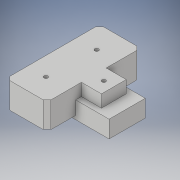
# Autodesk Inventor part: Connect_Male_Beauty
Saved by Autodesk Inventor 2019 (Build 230136000, 136)
## iProperties
Created: 2020-03-28
Part Number: Connect_Male_Beauty
Material: Generico
Document SubType Name: Modeling
Designer: Administrator
Density: 1 g/cm^3
Appearance: Default
Author: Administrator
Autodesk Inventor part; units mm, degrees
ref_plane "YZ Plane" through (0, 0, 0) normal (1, 0, 0) x (0, 1, 0)
ref_plane "XZ Plane" through (0, 0, 0) normal (0, 1, 0) x (-1, 0, 0)
ref_plane "XY Plane" through (0, 0, 0) normal (0, 0, 1) x (1, 0, 0)
sketch "Sketch1" plane through (0, 0, 0) normal (0, 1, 0) x (-1, 0, 0)
  line L0 (0, 0) -> (-17.5, 0)
  line L1 (-17.5, 0) -> (-17.5, -19)
  line L2 (-17.5, -19) -> (0, -19)
  line L3 (0, -19) -> (0, 0)
  dimension "d0" = 17.5
  dimension "d1" = 19
  constraints: 8 end point, 2 parallel, 1 horizontal, 1 perpendicular
  measures "d0" distance of L2.end L1.end
  measures "d1" distance of L1.end L0.end
extrude "Extrusion1" add sketch "Sketch1" along normal blind 9
sketch "Sketch2" plane through (0, 9, 0) normal (0, 1, 0) x (1, 0, 0)
  line L0 (0, 3) -> (10.5, 3)
  line L1 (10.5, 3) -> (10.5, 16)
  line L2 (10.5, 16) -> (0, 16)
  line L3 (0, 16) -> (0, 3)
  point P0 (0, 0)
  dimension "d4" = 10.5
  dimension "d5" = 13
  constraints: 8 end point, 2 parallel, 1 horizontal, 1 perpendicular
  measures "d4" distance of L2.end L1.end
  measures "d5" distance of L1.end L0.end
extrude "Extrusion2" add sketch "Sketch2" along normal blind 3
sketch "Sketch3" plane through (0, 0, -19) normal (-1, 0, 0) x (0, 0, 1)
  line L0 (18.2159, 3.93) -> (-8.9493, 3.93) construction
  line L1 (-8.9493, 3.93) -> (-8.9493, 7.5955) construction
  line L2 (-8.9493, 7.5955) -> (18.2159, 7.5955) construction
  line L3 (18.2159, 7.5955) -> (18.2159, 3.93) construction
  spline S0 degree 2 poles (15.88, 5.4433) (15.88, 5.6763) (15.9813, 6.1119) (16.0766, 6.2922) knots 0 0 0 1 2 2 2
  line L4 (16.0766, 6.2922) -> (16.6418, 6.2922)
  line L5 (16.6418, 6.2922) -> (16.6762, 6.0977)
  spline S1 degree 2 poles (16.6762, 6.0977) (16.7654, 6.1929) (16.9173, 6.3064) (17.049, 6.3064) knots 0 0 0 1 2 2 2
  spline S2 degree 2 poles (17.049, 6.3064) (17.2556, 6.3064) (17.519, 5.8911) (17.519, 5.498) knots 0 0 0 1 2 2 2
  spline S3 degree 2 poles (17.519, 5.498) (17.519, 5.103) (17.1949, 4.6634) (16.9882, 4.6634) knots 0 0 0 1 2 2 2
  spline S4 degree 2 poles (16.9882, 4.6634) (16.891, 4.6634) (16.7512, 4.7241) (16.6803, 4.7748) knots 0 0 0 1 2 2 2
  line L6 (16.6803, 4.7748) -> (16.6803, 4.6937)
  line L7 (16.6803, 4.6937) -> (16.4655, 4.6937)
  line L8 (16.4655, 4.6937) -> (16.4655, 6.1058)
  line L9 (16.4655, 6.1058) -> (16.1596, 6.1058)
  spline S5 degree 2 poles (16.1596, 6.1058) (16.109, 5.9863) (16.0644, 5.6074) (16.0644, 5.4535) knots 0 0 0 1 2 2 2
  spline S6 degree 2 poles (16.0644, 5.4535) (16.0644, 4.9044) (16.5121, 4.2359) (16.9315, 4.2359) knots 0 0 0 1 2 2 2
  spline S7 degree 2 poles (16.9315, 4.2359) (17.3286, 4.2359) (17.8472, 4.9591) (17.8472, 5.4758) knots 0 0 0 1 2 2 2
  spline S8 degree 2 poles (17.8472, 5.4758) (17.8472, 6.0288) (17.3448, 6.7156) (16.9396, 6.7156) knots 0 0 0 1 2 2 2
  spline S9 degree 2 poles (16.9396, 6.7156) (16.8302, 6.7156) (16.5891, 6.6792) (16.4817, 6.6386) knots 0 0 0 1 2 2 2
  line L10 (16.4817, 6.6386) -> (16.4817, 6.8757)
  spline S10 degree 2 poles (16.4817, 6.8757) (16.5952, 6.9101) (16.8282, 6.9364) (16.9396, 6.9364) knots 0 0 0 1 2 2 2
  spline S11 degree 2 poles (16.9396, 6.9364) (17.4157, 6.9364) (18.0397, 6.12) (18.0397, 5.4717) knots 0 0 0 1 2 2 2
  spline S12 degree 2 poles (18.0397, 5.4717) (18.0397, 4.8558) (17.3954, 4.009) (16.9335, 4.009) knots 0 0 0 1 2 2 2
  spline S13 degree 2 poles (16.9335, 4.009) (16.4392, 4.009) (15.88, 4.8052) (15.88, 5.4433) knots 0 0 0 1 2 2 2
  line L11 (16.6823, 5.8728) -> (16.6823, 5.0037)
  spline S14 degree 2 poles (16.6823, 5.0037) (16.7573, 4.9551) (16.8849, 4.9125) (16.9518, 4.9125) knots 0 0 0 1 2 2 2
  spline S15 degree 2 poles (16.9518, 4.9125) (17.1037, 4.9125) (17.2901, 5.1962) (17.2901, 5.494) knots 0 0 0 1 2 2 2
  spline S16 degree 2 poles (17.2901, 5.494) (17.2901, 5.7614) (17.1503, 6.0471) (16.9963, 6.0471) knots 0 0 0 1 2 2 2
  spline S17 degree 2 poles (16.9963, 6.0471) (16.9153, 6.0471) (16.7552, 5.9498) (16.6823, 5.8728) knots 0 0 0 1 2 2 2
  line L12 (15.7301, 6.5576) -> (15.0555, 4.0576)
  line L13 (15.0555, 4.0576) -> (14.7273, 4.0576)
  line L14 (14.7273, 4.0576) -> (14.0527, 6.5576)
  line L15 (14.0527, 6.5576) -> (14.3322, 6.5576)
  line L16 (14.3322, 6.5576) -> (14.5125, 5.8587)
  line L17 (14.5125, 5.8587) -> (15.2804, 5.8587)
  line L18 (15.2804, 5.8587) -> (15.4607, 6.5576)
  line L19 (15.4607, 6.5576) -> (15.7301, 6.5576)
  line L20 (14.5875, 5.575) -> (14.8975, 4.3919)
  line L21 (14.8975, 4.3919) -> (15.2054, 5.575)
  line L22 (15.2054, 5.575) -> (14.5875, 5.575)
  spline S18 degree 2 poles (13.1106, 5.9073) (13.1106, 6.2355) (13.4307, 6.592) (13.7022, 6.592) knots 0 0 0 1 2 2 2
  spline S19 degree 2 poles (13.7022, 6.592) (13.765, 6.592) (13.9817, 6.5637) (14.0547, 6.5434) knots 0 0 0 1 2 2 2
  line L23 (14.0547, 6.5434) -> (14.0547, 6.2233)
  line L24 (14.0547, 6.2233) -> (14.0405, 6.2233)
  spline S20 degree 2 poles (14.0405, 6.2233) (13.9838, 6.2476) (13.8217, 6.3044) (13.7366, 6.3044) knots 0 0 0 1 2 2 2
  spline S21 degree 2 poles (13.7366, 6.3044) (13.613, 6.3044) (13.4672, 6.2334) (13.4327, 6.1686) knots 0 0 0 1 2 2 2
  spline S22 degree 2 poles (13.4327, 6.1686) (13.3962, 6.1018) (13.376, 5.9073) (13.376, 5.7796) knots 0 0 0 1 2 2 2
  line L25 (13.376, 5.7796) -> (13.376, 4.323)
  line L26 (13.376, 4.323) -> (13.7994, 4.323)
  line L27 (13.7994, 4.323) -> (13.7994, 4.0576)
  line L28 (13.7994, 4.0576) -> (13.1106, 4.0576)
  line L29 (13.1106, 4.0576) -> (13.1106, 5.9073)
  spline S23 degree 2 poles (12.0206, 6.6103) (12.1969, 6.6103) (12.4603, 6.4948) (12.5535, 6.3793) knots 0 0 0 1 2 2 2
  spline S24 degree 2 poles (12.5535, 6.3793) (12.6588, 6.2497) (12.7439, 5.885) (12.7439, 5.6176) knots 0 0 0 1 2 2 2
  line L30 (12.7439, 5.6176) -> (12.7439, 4.0576)
  line L31 (12.7439, 4.0576) -> (12.4785, 4.0576)
  line L32 (12.4785, 4.0576) -> (12.4785, 5.6176)
  spline S25 degree 2 poles (12.4785, 5.6176) (12.4785, 5.7918) (12.4441, 6.0268) (12.3934, 6.122) knots 0 0 0 1 2 2 2
  spline S26 degree 2 poles (12.3934, 6.122) (12.3387, 6.2233) (12.1544, 6.3266) (12.0206, 6.3266) knots 0 0 0 1 2 2 2
  spline S27 degree 2 poles (12.0206, 6.3266) (11.8971, 6.3266) (11.7026, 6.2233) (11.6479, 6.122) knots 0 0 0 1 2 2 2
  spline S28 degree 2 poles (11.6479, 6.122) (11.5992, 6.0268) (11.5628, 5.7938) (11.5628, 5.6257) knots 0 0 0 1 2 2 2
  line L33 (11.5628, 5.6257) -> (11.5628, 4.0576)
  line L34 (11.5628, 4.0576) -> (11.2974, 4.0576)
  line L35 (11.2974, 4.0576) -> (11.2974, 5.6176)
  spline S29 degree 2 poles (11.2974, 5.6176) (11.2974, 5.8789) (11.3825, 6.2517) (11.4878, 6.3793) knots 0 0 0 1 2 2 2
  spline S30 degree 2 poles (11.4878, 6.3793) (11.583, 6.4968) (11.8363, 6.6103) (12.0206, 6.6103) knots 0 0 0 1 2 2 2
  spline S31 degree 2 poles (10.3594, 6.6022) (10.5762, 6.6022) (10.8821, 6.4887) (11.0158, 6.4077) knots 0 0 0 1 2 2 2
  line L36 (11.0158, 6.4077) -> (11.0158, 5.9903)
  line L37 (11.0158, 5.9903) -> (10.9975, 5.9903)
  spline S32 degree 2 poles (10.9975, 5.9903) (10.8659, 6.1443) (10.5316, 6.3145) (10.3776, 6.3145) knots 0 0 0 1 2 2 2
  spline S33 degree 2 poles (10.3776, 6.3145) (10.1568, 6.3145) (9.9319, 6.0856) (9.9319, 5.8971) knots 0 0 0 1 2 2 2
  spline S34 degree 2 poles (9.9319, 5.8971) (9.9319, 5.7472) (10.0514, 5.5608) (10.1791, 5.5142) knots 0 0 0 1 2 2 2
  spline S35 degree 2 poles (10.1791, 5.5142) (10.2723, 5.4818) (10.4262, 5.4373) (10.5417, 5.4008) knots 0 0 0 1 2 2 2
  spline S36 degree 2 poles (10.5417, 5.4008) (10.645, 5.3664) (10.8091, 5.263) (10.8719, 5.18) knots 0 0 0 1 2 2 2
  spline S37 degree 2 poles (10.8719, 5.18) (10.9327, 5.0969) (11.0016, 4.874) (11.0016, 4.7282) knots 0 0 0 1 2 2 2
  spline S38 degree 2 poles (11.0016, 4.7282) (11.0016, 4.4243) (10.6227, 4.013) (10.329, 4.013) knots 0 0 0 1 2 2 2
  spline S39 degree 2 poles (10.329, 4.013) (10.1608, 4.013) (9.861, 4.0961) (9.7334, 4.1751) knots 0 0 0 1 2 2 2
  line L38 (9.7334, 4.1751) -> (9.7334, 4.5722)
  line L39 (9.7334, 4.5722) -> (9.7536, 4.5722)
  spline S40 degree 2 poles (9.7536, 4.5722) (9.8488, 4.4628) (10.1467, 4.3007) (10.3108, 4.3007) knots 0 0 0 1 2 2 2
  spline S41 degree 2 poles (10.3108, 4.3007) (10.4971, 4.3007) (10.7261, 4.5175) (10.7261, 4.6937) knots 0 0 0 1 2 2 2
  spline S42 degree 2 poles (10.7261, 4.6937) (10.7261, 4.8518) (10.5903, 5.0402) (10.4627, 5.0827) knots 0 0 0 1 2 2 2
  spline S43 degree 2 poles (10.4627, 5.0827) (10.3796, 5.1111) (10.1345, 5.184) (10.0535, 5.2144) knots 0 0 0 1 2 2 2
  spline S44 degree 2 poles (10.0535, 5.2144) (9.8468, 5.2934) (9.6564, 5.6115) (9.6564, 5.8445) knots 0 0 0 1 2 2 2
  spline S45 degree 2 poles (9.6564, 5.8445) (9.6564, 5.9924) (9.7516, 6.276) (9.8367, 6.3753) knots 0 0 0 1 2 2 2
  spline S46 degree 2 poles (9.8367, 6.3753) (9.9339, 6.4847) (10.177, 6.6022) (10.3594, 6.6022) knots 0 0 0 1 2 2 2
  spline S47 degree 2 poles (8.1714, 5.6196) (8.1714, 6.0937) (8.536, 6.6103) (8.8399, 6.6103) knots 0 0 0 1 2 2 2
  spline S48 degree 2 poles (8.8399, 6.6103) (9.1519, 6.6103) (9.5105, 6.0775) (9.5105, 5.6196) knots 0 0 0 1 2 2 2
  spline S49 degree 2 poles (9.5105, 5.6196) (9.5105, 5.1496) (9.1418, 4.6289) (8.8399, 4.6289) knots 0 0 0 1 2 2 2
  spline S50 degree 2 poles (8.8399, 4.6289) (8.536, 4.6289) (8.1714, 5.1475) (8.1714, 5.6196) knots 0 0 0 1 2 2 2
  spline S51 degree 2 poles (8.4327, 5.6196) (8.4327, 5.2549) (8.6434, 4.9004) (8.8399, 4.9004) knots 0 0 0 1 2 2 2
  spline S52 degree 2 poles (8.8399, 4.9004) (9.0364, 4.9004) (9.2492, 5.2549) (9.2492, 5.6196) knots 0 0 0 1 2 2 2
  spline S53 degree 2 poles (9.2492, 5.6196) (9.2492, 5.9741) (9.0364, 6.3388) (8.8399, 6.3388) knots 0 0 0 1 2 2 2
  spline S54 degree 2 poles (8.8399, 6.3388) (8.6454, 6.3388) (8.4327, 5.9802) (8.4327, 5.6196) knots 0 0 0 1 2 2 2
  line L40 (7.124, 4.2501) -> (7.1381, 4.2501)
  spline S55 degree 2 poles (7.1381, 4.2501) (7.1706, 4.2339) (7.2962, 4.2055) (7.3468, 4.2055) knots 0 0 0 1 2 2 2
  spline S56 degree 2 poles (7.3468, 4.2055) (7.5048, 4.2055) (7.6406, 4.3838) (7.6406, 4.6188) knots 0 0 0 1 2 2 2
  line L41 (7.6406, 4.6188) -> (7.6406, 4.6816)
  line L42 (7.6406, 4.6816) -> (7.2253, 4.6816)
  line L43 (7.2253, 4.6816) -> (7.2253, 4.9429)
  line L44 (7.2253, 4.9429) -> (7.6325, 4.9429)
  line L45 (7.6325, 4.9429) -> (7.6325, 6.5576)
  line L46 (7.6325, 6.5576) -> (7.8857, 6.5576)
  line L47 (7.8857, 6.5576) -> (7.8857, 4.9429)
  line L48 (7.8857, 4.9429) -> (8.0559, 4.9429)
  line L49 (8.0559, 4.9429) -> (8.0559, 4.6816)
  line L50 (8.0559, 4.6816) -> (7.8857, 4.6816)
  line L51 (7.8857, 4.6816) -> (7.8857, 4.6188)
  spline S57 degree 2 poles (7.8857, 4.6188) (7.8857, 4.2825) (7.6264, 3.93) (7.3833, 3.93) knots 0 0 0 1 2 2 2
  spline S58 degree 2 poles (7.3833, 3.93) (7.3124, 3.93) (7.1787, 3.9482) (7.124, 3.9604) knots 0 0 0 1 2 2 2
  line L52 (7.124, 3.9604) -> (7.124, 4.2501)
  spline S59 degree 2 poles (6.583, 6.5941) (6.7897, 6.5941) (7.0206, 6.3003) (7.0206, 5.9822) knots 0 0 0 1 2 2 2
  line L53 (7.0206, 5.9822) -> (7.0206, 4.9429)
  line L54 (7.0206, 4.9429) -> (7.1908, 4.9429)
  line L55 (7.1908, 4.9429) -> (7.1908, 4.6816)
  line L56 (7.1908, 4.6816) -> (7.0206, 4.6816)
  line L57 (7.0206, 4.6816) -> (7.0206, 4.1427)
  line L58 (7.0206, 4.1427) -> (6.7674, 4.1427)
  line L59 (6.7674, 4.1427) -> (6.7674, 4.6816)
  line L60 (6.7674, 4.6816) -> (6.3035, 4.6816)
  line L61 (6.3035, 4.6816) -> (6.3035, 4.9429)
  line L62 (6.3035, 4.9429) -> (6.7674, 4.9429)
  line L63 (6.7674, 4.9429) -> (6.7674, 5.8364)
  spline S60 degree 2 poles (6.7674, 5.8364) (6.7674, 5.9782) (6.7593, 6.1342) (6.733, 6.201) knots 0 0 0 1 2 2 2
  spline S61 degree 2 poles (6.733, 6.201) (6.7107, 6.2598) (6.6074, 6.3185) (6.5202, 6.3185) knots 0 0 0 1 2 2 2
  spline S62 degree 2 poles (6.5202, 6.3185) (6.4595, 6.3185) (6.344, 6.2719) (6.3176, 6.2578) knots 0 0 0 1 2 2 2
  line L64 (6.3176, 6.2578) -> (6.3035, 6.2578)
  line L65 (6.3035, 6.2578) -> (6.3035, 6.5414)
  spline S63 degree 2 poles (6.3035, 6.5414) (6.3744, 6.5657) (6.5202, 6.5941) (6.583, 6.5941) knots 0 0 0 1 2 2 2
  line L66 (5.724, 6.5576) -> (6.0441, 6.5576)
  line L67 (6.0441, 6.5576) -> (6.0441, 6.0795)
  line L68 (6.0441, 6.0795) -> (5.724, 6.0795)
  line L69 (5.724, 6.0795) -> (5.724, 6.5576)
  spline S64 degree 2 poles (4.6888, 6.6001) (4.8428, 6.6001) (5.1001, 6.4806) (5.1933, 6.3591) knots 0 0 0 1 2 2 2
  spline S65 degree 2 poles (5.1933, 6.3591) (5.2864, 6.2395) (5.3877, 5.8708) (5.3877, 5.6236) knots 0 0 0 1 2 2 2
  spline S66 degree 2 poles (5.3877, 5.6236) (5.3877, 5.3765) (5.2824, 5.0159) (5.1933, 4.8943) knots 0 0 0 1 2 2 2
  spline S67 degree 2 poles (5.1933, 4.8943) (5.1041, 4.7707) (4.8407, 4.639) (4.6888, 4.639) knots 0 0 0 1 2 2 2
  spline S68 degree 2 poles (4.6888, 4.639) (4.5652, 4.639) (4.3343, 4.7262) (4.2451, 4.7829) knots 0 0 0 1 2 2 2
  line L70 (4.2451, 4.7829) -> (4.2451, 5.1374)
  line L71 (4.2451, 5.1374) -> (4.2593, 5.1374)
  spline S69 degree 2 poles (4.2593, 5.1374) (4.2877, 5.1091) (4.3707, 5.0361) (4.4315, 4.9976) knots 0 0 0 1 2 2 2
  spline S70 degree 2 poles (4.4315, 4.9976) (4.4842, 4.9652) (4.626, 4.9146) (4.6928, 4.9146) knots 0 0 0 1 2 2 2
  spline S71 degree 2 poles (4.6928, 4.9146) (4.8894, 4.9146) (5.1264, 5.2853) (5.1264, 5.6236) knots 0 0 0 1 2 2 2
  spline S72 degree 2 poles (5.1264, 5.6236) (5.1264, 5.9539) (4.8975, 6.3246) (4.6928, 6.3246) knots 0 0 0 1 2 2 2
  spline S73 degree 2 poles (4.6928, 6.3246) (4.5693, 6.3246) (4.3464, 6.197) (4.2593, 6.0977) knots 0 0 0 1 2 2 2
  line L72 (4.2593, 6.0977) -> (4.2451, 6.0977)
  line L73 (4.2451, 6.0977) -> (4.2451, 6.4522)
  spline S74 degree 2 poles (4.2451, 6.4522) (4.2836, 6.4745) (4.395, 6.5373) (4.4416, 6.5515) knots 0 0 0 1 2 2 2
  spline S75 degree 2 poles (4.4416, 6.5515) (4.5065, 6.5758) (4.6078, 6.6001) (4.6888, 6.6001) knots 0 0 0 1 2 2 2
  spline S76 degree 2 poles (2.7824, 5.6196) (2.7824, 6.0937) (3.1471, 6.6103) (3.4509, 6.6103) knots 0 0 0 1 2 2 2
  spline S77 degree 2 poles (3.4509, 6.6103) (3.7629, 6.6103) (4.1215, 6.0775) (4.1215, 5.6196) knots 0 0 0 1 2 2 2
  spline S78 degree 2 poles (4.1215, 5.6196) (4.1215, 5.1496) (3.7528, 4.6289) (3.4509, 4.6289) knots 0 0 0 1 2 2 2
  spline S79 degree 2 poles (3.4509, 4.6289) (3.1471, 4.6289) (2.7824, 5.1475) (2.7824, 5.6196) knots 0 0 0 1 2 2 2
  spline S80 degree 2 poles (3.0437, 5.6196) (3.0437, 5.2549) (3.2544, 4.9004) (3.4509, 4.9004) knots 0 0 0 1 2 2 2
  spline S81 degree 2 poles (3.4509, 4.9004) (3.6475, 4.9004) (3.8602, 5.2549) (3.8602, 5.6196) knots 0 0 0 1 2 2 2
  spline S82 degree 2 poles (3.8602, 5.6196) (3.8602, 5.9741) (3.6475, 6.3388) (3.4509, 6.3388) knots 0 0 0 1 2 2 2
  spline S83 degree 2 poles (3.4509, 6.3388) (3.2565, 6.3388) (3.0437, 5.9802) (3.0437, 5.6196) knots 0 0 0 1 2 2 2
  line L74 (0.8213, 6.5576) -> (0.8213, 5.4717)
  spline S84 degree 2 poles (0.8213, 5.4717) (0.8213, 5.342) (0.8375, 5.1212) (0.8618, 5.0604) knots 0 0 0 1 2 2 2
  spline S85 degree 2 poles (0.8618, 5.0604) (0.8902, 4.9936) (0.9894, 4.9287) (1.0725, 4.9287) knots 0 0 0 1 2 2 2
  spline S86 degree 2 poles (1.0725, 4.9287) (1.1515, 4.9287) (1.3298, 5.0483) (1.425, 5.1617) knots 0 0 0 1 2 2 2
  spline S87 degree 2 poles (1.425, 5.1617) (1.423, 5.1901) (1.4189, 5.2691) (1.4189, 5.3218) knots 0 0 0 1 2 2 2
  line L75 (1.4189, 5.3218) -> (1.4189, 6.5576)
  line L76 (1.4189, 6.5576) -> (1.6722, 6.5576)
  line L77 (1.6722, 6.5576) -> (1.6722, 5.4717)
  spline S88 degree 2 poles (1.6722, 5.4717) (1.6722, 5.342) (1.6884, 5.1212) (1.7127, 5.0604) knots 0 0 0 1 2 2 2
  spline S89 degree 2 poles (1.7127, 5.0604) (1.7411, 4.9936) (1.8403, 4.9287) (1.9234, 4.9287) knots 0 0 0 1 2 2 2
  spline S90 degree 2 poles (1.9234, 4.9287) (2.0065, 4.9287) (2.1847, 5.0564) (2.2698, 5.1557) knots 0 0 0 1 2 2 2
  line L78 (2.2698, 5.1557) -> (2.2698, 6.5576)
  line L79 (2.2698, 6.5576) -> (2.5231, 6.5576)
  line L80 (2.5231, 6.5576) -> (2.5231, 4.6816)
  line L81 (2.5231, 4.6816) -> (2.2698, 4.6816)
  line L82 (2.2698, 4.6816) -> (2.2698, 4.8882)
  spline S91 degree 2 poles (2.2698, 4.8882) (2.1706, 4.7646) (1.9761, 4.6289) (1.8586, 4.6289) knots 0 0 0 1 2 2 2
  spline S92 degree 2 poles (1.8586, 4.6289) (1.7269, 4.6289) (1.5202, 4.7809) (1.4676, 4.9531) knots 0 0 0 1 2 2 2
  spline S93 degree 2 poles (1.4676, 4.9531) (1.3541, 4.793) (1.1353, 4.6289) (1.0077, 4.6289) knots 0 0 0 1 2 2 2
  spline S94 degree 2 poles (1.0077, 4.6289) (0.9125, 4.6289) (0.7524, 4.7039) (0.6937, 4.789) knots 0 0 0 1 2 2 2
  spline S95 degree 2 poles (0.6937, 4.789) (0.6329, 4.874) (0.568, 5.1293) (0.568, 5.3218) knots 0 0 0 1 2 2 2
  line L83 (0.568, 5.3218) -> (0.568, 6.5576)
  line L84 (0.568, 6.5576) -> (0.8213, 6.5576)
  point P0 (19, 0)
  constraints: 2 other
extrude "Extrusion3" cut sketch "Sketch3" against normal blind 1
sketch "Sketch4" plane through (0, 0, -19) normal (-1, 0, 0) x (0, 0, 1)
  line L0 (0.4166, 8.6289) -> (18.4748, 8.6289)
  line L1 (18.4748, 8.6289) -> (18.4748, 1.9759)
  line L2 (18.4748, 1.9759) -> (0.4166, 1.9759)
  line L3 (0.4166, 1.9759) -> (0.4166, 8.6289)
  point P0 (19, 0)
  constraints: 8 end point, 2 parallel, 1 horizontal, 1 perpendicular
extrude "Extrusion4" add sketch "Sketch4" against normal blind 10
sketch "Sketch5" plane through (0, 0, -19) normal (-1, 0, 0) x (0, 0, 1)
  line L0 (-15, 9) -> (34, 9)
  line L1 (34, 9) -> (34, 0)
  line L2 (34, 0) -> (-15, 0)
  line L3 (-15, 0) -> (-15, 9)
  point P0 (19, 0)
  dimension "d12" = 49
  constraints: 8 end point, 2 parallel, 1 horizontal, 1 perpendicular
  measures "d12" distance of L1.end L2.end
extrude "Extrusion5" add sketch "Sketch5" along normal blind 15
move faces "Move1" translate (-6.5, 0, 0) faces at (-15, 6, -17.6667)
sketch "Sketch6" plane through (0, 0, 0) normal (0, -1, 0) x (1, 0, 0)
  line L0 (17.5, 0) -> (17.5, -19) projected
  line L1 (17.5, -19) -> (0, -19) projected
  line L2 (17.5, 0) -> (0, -19)
  line L3 (0, -16) -> (0, -3) projected
  line L4 (0, 15) -> (-21.5, 15) projected
  line L5 (0, -9.5) -> (-21.5, 15)
  line L6 (-21.5, -34) -> (-21.5, 15) projected
  line L7 (0, -9.5) -> (-21.5, -34)
  circle A0 centre (-10.75, -21.75) radius 1
  circle A1 centre (-10.75, 2.75) radius 1
  circle A2 centre (8.75, -9.5) radius 1
  point P0 (0, 0)
  dimension "d18" = 2
  dimension "d19" = 2
  dimension "d20" = 2
  constraints: 6 end point, 4 midpoint, 3 centre point
  measures "d18" diameter of A0
  measures "d19" diameter of A1
  measures "d20" diameter of A2
extrude "Extrusion6" cut sketch "Sketch6" against normal blind 3 contours A2 L2 | L2 A2 | A1 L5 | L5 A1 | A0 L7 | L7 A0
sketch "Sketch7" plane through (8.75, 3, -9.5) normal (0, -1, 0) x (1, 0, 0)
  circle A0 centre (0, 0) radius 0.5
  circle A1 centre (-19.5, 12.25) radius 1 projected
  circle A2 centre (-19.5, 12.25) radius 0.5
  circle A3 centre (-19.5, -12.25) radius 1 projected
  circle A4 centre (-19.5, -12.25) radius 0.5
  point P0 (-8.75, 9.5)
  dimension "d23" = 1
  dimension "d24" = 1
  dimension "d25" = 1
  constraints: 3 centre point, 2 coincident
  measures "d23" diameter of A0
  measures "d24" diameter of A2
  measures "d25" diameter of A4
extrude "Extrusion7" cut sketch "Sketch7" against normal blind 3 contours A0 | A2 | A4
sketch "Sketch8" plane through (0, 9, 0) normal (0, 1, 0) x (1, 0, 0)
  line L0 (0, 34) -> (-21.5, 34) projected
  line L1 (-21.5, 34) -> (-21.5, -15) projected
  line L2 (0, 34) -> (-21.5, 34)
  line L3 (-21.5, 34) -> (-21.5, -15)
  line L4 (-21.5, -15) -> (0, -15)
  line L5 (0, -15) -> (0, 34)
  point P0 (0, 16)
  constraints: 8 end point, 2 parallel, 1 horizontal, 1 perpendicular
sketch "Sketch9" plane through (0, 0, 0) normal (0, -1, 0) x (1, 0, 0)
  line L0 (12.3887, -6.6265) -> (12.3887, -13.157)
  line L1 (12.3887, -13.157) -> (-3.9375, -13.157)
  line L2 (-3.9375, -13.157) -> (-3.9375, -28.5228)
  line L3 (-3.9375, -28.5228) -> (-15.6539, -28.5228)
  line L4 (-15.6539, -28.5228) -> (-15.6539, 8.3552)
  line L5 (-15.6539, 8.3552) -> (-3.9375, 8.3552)
  line L6 (-3.9375, 8.3552) -> (-3.9375, -6.6265)
  line L7 (-3.9375, -6.6265) -> (12.3887, -6.6265)
  point P0 (0, 0)
  constraints: 16 end point, 6 perpendicular, 2 point on line, 1 vertical
extrude "Extrusion8" add sketch "Sketch9" against normal blind 6
extrude "Extrusion9" add sketch "Sketch8" along normal blind 3
move faces "Move2" translate (0, 3.5, 0) faces at (-14.3333, 12, -11.6667)
sketch "Sketch10" plane through (-21.5, 15.5, -34) normal (0, 1, 0) x (1, 0, 0)
  line L0 (32, -18) -> (32, -31) projected
  line L1 (21.5, -31) -> (21.5, -34) projected
  line L2 (32, -18) -> (21.5, -31)
  line L3 (21.5, -31) -> (21.5, -18)
  line L4 (0, 0) -> (0, -49) projected
  line L5 (21.5, -24.5) -> (0, 0)
  line L6 (21.5, -24.5) -> (0, -49)
  circle A0 centre (10.75, -12.25) radius 1
  circle A1 centre (9.75, -37.8895) radius 1
  circle A2 centre (26.75, -24.5) radius 1
  dimension "d36" = 2
  dimension "d37" = 2
  dimension "d38" = 2
  constraints: 8 end point, 3 centre point, 3 midpoint, 1 collinear, 1 point on line
  measures "d36" diameter of A0
  measures "d37" diameter of A1
  measures "d38" diameter of A2
extrude "Extrusion10" cut sketch "Sketch10" against normal blind 3 contours A2 L2 | L2 A2 | A0 L5 | L5 A0 | A1 L6 | L6 A1
sketch "Sketch11" plane through (5.25, 12.5, -9.5) normal (0, 1, 0) x (1, 0, 0)
  circle A0 centre (0, 0) radius 1 projected
  circle A1 centre (0, 0) radius 0.5
  circle A2 centre (-16, 12.25) radius 1 projected
  circle A3 centre (-16, 12.25) radius 0.5
  circle A4 centre (-17, -13.3895) radius 1 projected
  circle A5 centre (-17, -13.3895) radius 0.5
  point P0 (-5.25, -9.5)
  dimension "d41" = 1
  dimension "d42" = 1
  dimension "d43" = 1
  constraints: 3 centre point, 3 coincident
  measures "d41" diameter of A1
  measures "d42" diameter of A3
  measures "d43" diameter of A5
extrude "Extrusion11" cut sketch "Sketch11" against normal blind 3 contours A1 | A3 | A5
chamfer "Chamfer1" distance 2 angle 45 5 edges at (-21.5, 0, -9.5) (-10.75, 0, -34) (0, 0, -26.5) (0, 0, 7.5) (-10.75, 0, 15)
chamfer "Chamfer2" distance 2 angle 45 8 edges at (-20.5, 1, -33) (-21.5, 8.75, -34) (0, 8.75, -34) (-1, 1, -33) (-1, 1, 14) (0, 8.75, 15) (-20.5, 1, 14) (-21.5, 8.75, 15)
body "Solid1"
